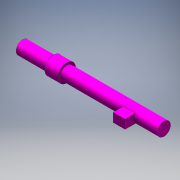
# Autodesk Inventor part: battery gate pin
Saved by Autodesk Inventor 2016 (Build 200138000, 138)
## iProperties
Created: 2015-09-29
Part Number: battery gate pin
Material: Generic
Document SubType Name: Modeling
Designer: Hulbert Office
Density: 1 g/cm^3
Appearance: Default
Author: Hulbert Office
Autodesk Inventor part; units mm, degrees
ref_plane "YZ Plane" through (0, 0, 0) normal (1, 0, 0) x (0, 1, 0)
ref_plane "XY Plane" through (0, 0, 0) normal (0, 0, 1) x (1, 0, 0)
sketch "Sketch1" plane through (0, 0, 0) normal (1, 0, 0) x (0, 1, 0)
  circle A0 centre (0, 0) radius 1.5
  dimension "d0" = 3
  constraints: 1 centre point, 1 coincident
  measures "d0" diameter of A0
extrude "Extrusion1" add sketch "Sketch1" along normal blind 7
sketch "Sketch2" plane through (7, 0, 0) normal (1, 0, 0) x (0, 0, -1)
  circle A0 centre (0, 0) radius 2
  dimension "d3" = 4
  constraints: 1 centre point, 1 coincident
  measures "d3" diameter of A0
extrude "Extrusion2" add sketch "Sketch2" along normal blind 3
sketch "Sketch3" plane through (10, 0, 0) normal (1, 0, 0) x (0, 0, -1)
  circle A0 centre (0, 0) radius 1.5
  dimension "d6" = 3
  constraints: 1 centre point, 1 coincident
  measures "d6" diameter of A0
extrude "Extrusion3" add sketch "Sketch3" along normal blind 22
ref_plane "Work Plane1" through (0, -1.5, 0) normal (0, 1, 0) x (-1, 0, 0)
sketch "Sketch6" plane through (0, -1.5, 0) normal (0, 1, 0) x (-1, 0, 0)
  line L0 (-32, 1.5) -> (-32, -1.5) projected
  line L1 (-32, 0) -> (-24, 0)
  line L2 (-10, -1.5) -> (-32, -1.5) projected
  line L3 (-24, 0) -> (-24, -1)
  line L4 (-24, 0) -> (-24, 1)
  line L5 (-24, 1) -> (-26.7, 1)
  line L6 (-26.7, 1) -> (-26.7, -1)
  line L7 (-26.7, -1) -> (-24, -1)
  point P0 (0, 0)
  dimension "d13" = 8
  dimension "d14" = 1
  dimension "d15" = 1
  dimension "d16" = 2.7
  constraints: 12 end point, 2 horizontal, 2 perpendicular, 2 vertical, 1 midpoint
  measures "d13" distance of L1.start L1.end
  measures "d14" distance of L1.end L3.end
  measures "d15" distance of L1.end L4.end
  measures "d16" distance of L4.end L5.end
extrude "Extrusion5" add sketch "Sketch6" against normal blind 2
extrude "Extrusion6" add sketch "Sketch6" along normal blind 1
body "Solid1"
